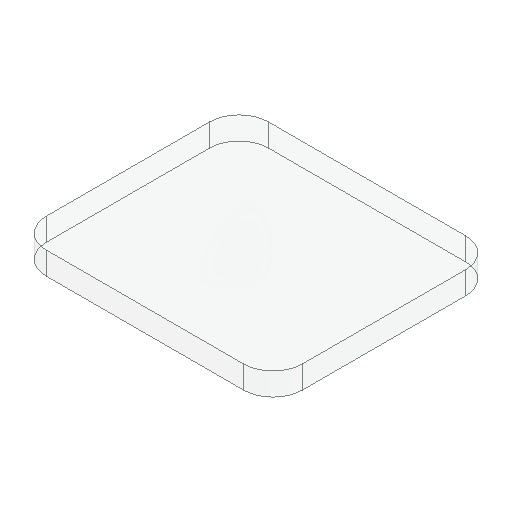
# Autodesk Inventor part: plexiglas_4mm
Saved by Autodesk Inventor 2025 (Build 290162000, 162)
## iProperties
Created: 2025-01-02
Part Number: plexiglas_4mm
Material: Glass
Document SubType Name: Modeling
Designer: Jan Mareš
Density: 2.18 g/cm^3
Appearance: Clear
Author: Jan Mareš
Autodesk Inventor part; units mm, degrees
ref_plane "YZ Plane" through (0, 0, 0) normal (1, 0, 0) x (0, 1, 0)
ref_plane "XZ Plane" through (0, 0, 0) normal (0, 1, 0) x (-1, 0, 0)
ref_plane "XY Plane" through (0, 0, 0) normal (0, 0, 1) x (1, 0, 0)
sketch "Sketch1" plane through (0, 0, 0) normal (0, 1, 0) x (-1, 0, 0)
  line L0 (31.64, 0) -> (-31.64, 0) construction
  line L1 (0, -27.44) -> (0, 27.44) construction
  line L2 (-22.6, 19.6) -> (22.6, 19.6)
  line L3 (22.6, 19.6) -> (22.6, -19.6)
  line L4 (22.6, -19.6) -> (-22.6, -19.6)
  line L5 (-22.6, -19.6) -> (-22.6, 19.6)
  line L6 (-22.6, 0) -> (22.6, 0) construction
  point P0 (0, 0)
  dimension "d0" = 45.2
  dimension "d1" = 39.2
  constraints: 10 end point, 3 midpoint, 2 parallel, 1 horizontal, 1 perpendicular
  measures "d0" distance of L2.start L2.end
  measures "d1" distance of L4.end L2.start
extrude "Extrusion1" add sketch "Sketch1" along normal blind 4
fillet "Fillet1" radius 5.2 4 edges at (-22.6, 2, 19.6) (22.6, 2, 19.6) (22.6, 2, -19.6) (-22.6, 2, -19.6)
body "Solid1"
